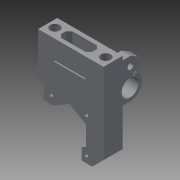
# Autodesk Inventor part: x-end-motor
Saved by Autodesk Inventor 2015 (Build 190159000, 159)
## iProperties
Created: 2015-06-01
Part Number: x-end-motor
Material: Generic
Document SubType Name: Modeling
Designer: X
Density: 1 g/cm^3
Appearance: Default
Author: X
Autodesk Inventor part; units mm, degrees
ref_plane "YZ Plane" through (0, 0, 0) normal (1, 0, 0) x (0, 1, 0)
ref_plane "XZ Plane" through (0, 0, 0) normal (0, 1, 0) x (-1, 0, 0)
ref_plane "XY Plane" through (0, 0, 0) normal (0, 0, 1) x (1, 0, 0)
sketch "Sketch1" plane through (0, 0, 0) normal (0, 1, 0) x (-1, 0, 0)
  line L0 (0, 0) -> (58, 0)
  line L1 (58, 0) -> (58, -81.5)
  line L2 (58, -81.5) -> (0, -81.5)
  line L3 (0, -81.5) -> (0, 0)
  dimension "d0" = 81.5
  dimension "d1" = 58
  constraints: 8 end point, 2 parallel, 1 horizontal, 1 perpendicular
  measures "d0" distance of L0.end L1.end
  measures "d1" distance between parallel lines of L3 L1
extrude "Extrusion1" add sketch "Sketch1" along normal blind 35
sketch "Sketch2" plane through (0, 35, 0) normal (0, 1, 0) x (1, 0, 0)
  line L0 (-30.25, 43.5) -> (-44.9724, 52)
  line L1 (-44.9724, 52) -> (-44.9724, 69)
  line L2 (-44.9724, 69) -> (-30.25, 77.5)
  line L3 (-30.25, 77.5) -> (-15.5276, 69)
  line L4 (-15.5276, 69) -> (-15.5276, 52)
  line L5 (-15.5276, 52) -> (-30.25, 43.5)
  line L6 (-58, 81.5) -> (-58, 0) projected
  line L7 (0, 81.5) -> (-58, 81.5) projected
  line L8 (-44.9724, 52) -> (-53, 52)
  line L9 (-19.25, 81.5) -> (-19.25, 71.1491)
  line L10 (0, 0) -> (0, 81.5) projected
  line L11 (-53, 52) -> (-53, 39.5)
  line L12 (-53, 39.5) -> (-58, 39.5)
  line L13 (-58, 39.5) -> (-58, 81.5)
  point P0 (-30.25, 60.5)
  dimension "d4" = 17
  dimension "d5" = 38
  dimension "d6" = 27.75
  dimension "d7" = 19.25
  dimension "d24" = 12.5
  dimension "d25" = 5
  constraints: 22 end point, 3 point on line, 2 perpendicular, 2 vertical, 1 parallel, 13 other
  measures "d4" distance of L3.end L4.end
  measures "d5" distance from line of L7 L0.start
  measures "d6" distance from line of L6 L0.start
  measures "d7" distance between parallel lines of L10 L9
  measures "d24" distance of L8.end L11.end
  measures "d25" distance of L11.end L12.end
extrude "Extrusion2" cut sketch "Sketch2" against normal through all
sketch "Sketch3" plane through (0, 0, 0) normal (1, 0, 0) x (0, 0, -1)
  line L0 (81.5, 0) -> (0, 0)
  line L1 (0, 0) -> (0, 17)
  line L2 (81.5, 17) -> (81.5, 0)
  line L3 (0, 0) -> (0, 35) projected
  line L4 (15.5, 30.8564) -> (19.5, 23.9282)
  line L5 (15.5, 17) -> (7.5, 17)
  line L6 (3.5, 23.9282) -> (7.5, 30.8564)
  line L7 (7.5, 30.8564) -> (15.5, 30.8564)
  line L8 (3.5, 23.9282) -> (3.5, 17)
  line L9 (19.5, 23.9282) -> (19.5, 17)
  circle A0 centre (27.7462, 23.5) radius 7.5
  circle A1 centre (27.7462, 23.5) radius 10.5
  line L10 (38.2462, 23.5) -> (38.2462, 17)
  line L11 (0, 17) -> (24.0046, 17)
  line L12 (31.4879, 17) -> (81.5, 17)
  point P0 (11.5, 23.9282)
  dimension "d10" = 17
  dimension "d11" = 3
  dimension "d12" = 15
  dimension "d13" = 6.5
  dimension "d14" = 3.5
  dimension "d15" = 8
  constraints: 24 end point, 7 perpendicular, 4 point on circle, 3 collinear, 3 parallel, 3 point on line, 2 centre point, 1 horizontal, 1 tangent, 9 other
  measures "d10" distance of L2.start L0.start
  measures "d11" radial gap between concentric circles of A1 A0
  measures "d12" diameter of A0
  measures "d13" distance of L10.start L10.end
  measures "d14" distance between parallel lines of L3 L8
  measures "d15" distance of L6.end L4.start
extrude "Extrusion4" cut sketch "Sketch3" against normal through all contours L0 L1 L11 L5 A1 L12 L2 | L12 A1 L10 | L8 L6 L7 L4 A1 L11 L5 | A1 L12 A0 L11 L9 L4 | A1 L11 A0 L12 | L4 L9 A1 keep common part
sketch "Sketch4" plane through (-58, 0, 0) normal (0, 0, 1) x (1, 0, 0)
  line L0 (0, 17) -> (50, 17)
  line L1 (50, 17) -> (50, 30.8564)
  line L2 (50, 30.8564) -> (0, 30.8564)
  line L3 (0, 30.8564) -> (0, 17)
  line L4 (0, 17) -> (58, 17) projected
  line L5 (0, 0) -> (0, 17) projected
  line L6 (58, 17) -> (58, 23.9282) projected
  line L7 (58, 30.8564) -> (0, 30.8564) projected
  point P0 (58, 0)
  point P1 (0, 35)
  dimension "d21" = 8
  constraints: 8 end point, 3 collinear, 2 parallel, 1 horizontal, 1 perpendicular
  measures "d21" distance between parallel lines of L6 L1
extrude "Extrusion5" cut sketch "Sketch4" against normal up to surface (17.8017 mm away)
sketch "Sketch5" plane through (0, 17, -38.2462) normal (0, 1, 0) x (1, 0, 0)
  line L0 (-8, -20.4446) -> (-58, -20.4446) projected
  line L1 (-16, -20.4446) -> (-44, -20.4446)
  line L2 (-44, -20.4446) -> (-44, -21.4446)
  line L3 (-44, -21.4446) -> (-16, -21.4446)
  line L4 (-16, -21.4446) -> (-16, -20.4446)
  line L5 (-8, -20.4446) -> (-8, -22.7462) projected
  point P0 (0, -38.2462)
  dimension "d26" = 8
  dimension "d27" = 1
  dimension "d28" = 28
  constraints: 8 end point, 2 parallel, 1 horizontal, 1 perpendicular, 1 point on line
  measures "d26" distance between parallel lines of L5 L4
  measures "d27" distance of L1.end L2.end
  measures "d28" distance of L2.end L3.end
extrude "Extrusion6" cut sketch "Sketch5" against normal through all
sketch "Sketch6" plane through (-44.9724, 0, -52) normal (0, 0, -1) x (-1, 0, 0)
  line L0 (-25.7224, 13.5) -> (-3.7224, 13.5)
  line L1 (-3.7224, 13.5) -> (-3.7224, 3.5)
  line L2 (-3.7224, 3.5) -> (-25.7224, 3.5)
  line L3 (-25.7224, 3.5) -> (-25.7224, 13.5)
  line L4 (-14.7224, 17) -> (-14.7224, 0) projected
  line L5 (-25.7224, 13.5) -> (-3.7224, 3.5) construction
  line L6 (-3.7224, 13.5) -> (-25.7224, 3.5) construction
  point P0 (-44.9724, 0)
  point P1 (-14.7224, 8.5)
  point P2 (-14.7224, 35)
  dimension "d31" = 10
  dimension "d32" = 22
  constraints: 12 end point, 3 midpoint, 2 parallel, 1 horizontal, 1 perpendicular
  measures "d31" distance of L0.end L1.end
  measures "d32" distance of L1.end L2.end
extrude "Extrusion7" cut sketch "Sketch6" against normal through all
sketch "Sketch7" plane through (-58, 0, 0) normal (0, 0, 1) x (1, 0, 0)
  line L0 (38.75, 3.5) -> (41.5, 6.25)
  line L1 (41.5, 6.25) -> (41.5, 10.75)
  line L2 (41.5, 10.75) -> (38.75, 13.5)
  line L3 (27.75, 3.5) -> (27.75, 13.5) construction
  line L4 (16.75, 13.5) -> (38.75, 13.5) construction
  line L5 (38.75, 13.5) -> (27.75, 13.5)
  line L6 (38.75, 3.5) -> (27.75, 3.5)
  line L7 (16.75, 3.5) -> (38.75, 3.5) projected
  line L8 (27.75, 8.5) -> (41.5, 8.5) construction
  line L9 (16.75, 3.5) -> (14, 6.25)
  line L10 (14, 6.25) -> (14, 10.75)
  line L11 (14, 10.75) -> (16.75, 13.5)
  line L12 (38.75, 13.5) -> (16.75, 13.5) construction
  line L13 (16.75, 13.5) -> (27.75, 13.5)
  line L14 (16.75, 3.5) -> (27.75, 3.5)
  point P0 (58, 0)
  dimension "d39" = 13.75
  dimension "d40" = 135
  dimension "d41" = 2.75
  constraints: 26 end point, 5 symmetric about line, 3 midpoint, 2 collinear, 2 point on line, 1 perpendicular, 1 other
  measures "d39" distance between parallel lines of L1 L3
  measures "d40" angle of L0 L6
  measures "d41" distance from line of L1 L0.start
extrude "Extrusion9" cut sketch "Sketch7" against normal blind 41.5
sketch "Sketch8" plane through (0, 17, -38.2462) normal (0, 1, 0) x (1, 0, 0)
  line L0 (-46.515, 6.0938) -> (-15.515, 6.0938) construction
  line L1 (-15.515, 6.0938) -> (-15.515, 37.0938) construction
  line L2 (-53, 13.7538) -> (-53, 1.2538) construction
  line L3 (-44.9724, 13.7538) -> (-53, 13.7538) construction
  point P0 (0, -38.2462)
  dimension "d45" = 31
  dimension "d46" = 31
  dimension "d47" = 6.485
  dimension "d48" = 7.66
  constraints: 4 end point, 1 horizontal, 1 perpendicular
  measures "d45" distance of L0.start L0.end
  measures "d46" distance of L1.end L0.end
  measures "d47" distance from line of L2 L0.start
  measures "d48" distance from line of L3 L0.start
hole "Hole1" at (-46.515, 17, -44.34) at (-15.515, 17, -44.34) at (-15.515, 17, -75.34) direction (0, -1, 0) diameter 3.6 end through all counterbore diameter 6.2 counterbore depth 3.5
sketch "Sketch9" plane through (-58, 0, 0) normal (0, 0, 1) x (1, 0, 0)
  line L0 (0, 0) -> (0, 17) construction
  line L1 (0, 8.5) -> (58, 8.5) construction
  line L2 (58, 0) -> (58, 17) construction
  line L3 (58, 0) -> (0, 0) construction
  point P0 (51.5, 8.5)
  point P1 (6.5, 8.5)
  point P2 (0, 35)
  point P3 (58, 35)
  dimension "d56" = 45
  dimension "d57" = 8.5
  dimension "d58" = 6.5
  constraints: 2 end point, 2 midpoint, 2 point on line, 1 horizontal
  measures "d56" distance of point (51.5, 8.5) point (6.5, 8.5)
  measures "d57" distance between parallel lines of L3 L1
  measures "d58" distance from line of L0 point (6.5, 8.5)
hole "Hole2" at (-6.5, 8.5, 0) at (-51.5, 8.5, 0) direction (0, 0, -1) diameter 8.5 depth 37
chamfer "Chamfer1" distance 10 angle 45 1 edges at (0, 8.5, -81.5)
hole "Hole3" at (0, 23.9282, -11.5) direction (-1, 0, 0) diameter 5.4 end through all
sketch "Sketch12" plane through (-8, 17, -17.8017) normal (-1, 0, 0) x (0, 0, 1)
  line L0 (8.5517, 10.8252) -> (10.8017, 6.9282)
  line L1 (10.8017, 6.9282) -> (8.5517, 3.0312)
  line L2 (8.5517, 3.0312) -> (4.0519, 3.0312)
  line L3 (4.0519, 3.0312) -> (1.8019, 6.9282)
  line L4 (1.8019, 6.9282) -> (4.0519, 10.8252)
  line L5 (4.0519, 10.8252) -> (8.5517, 10.8252)
  line L6 (2.3017, 13.8564) -> (10.3017, 13.8564) projected
  line L7 (10.3017, 13.8564) -> (14.3017, 6.9282) projected
  line L8 (10.8017, 6.9282) -> (14.3017, 6.9282) construction
  point P0 (17.8017, -17)
  point P1 (6.3018, 6.9282)
  dimension "d77" = 3.5
  dimension "d78" = 7.794
  constraints: 14 end point, 2 parallel, 1 horizontal, 13 other
  measures "d77" distance of L7.end L0.end
  measures "d78" distance between parallel lines of L2 L5
extrude "Extrusion10" cut sketch "Sketch12" against normal blind 5
sketch "Sketch13" plane through (-58, 0, -39.5) normal (-1, 0, 0) x (0, 0, 1)
  circle A0 centre (11.7538, 23.5) radius 7.5 projected
  line L0 (21.6983, 26.8698) -> (24, 30.8564) projected
  line L1 (18.874, 25.8564) -> (18.4972, 26.7827)
  line L2 (18.4972, 26.7827) -> (22.6151, 28.4577)
  line L3 (22.6151, 28.4577) -> (22.9919, 27.5314)
  line L4 (22.9919, 27.5314) -> (18.874, 25.8564)
  point P0 (39.5, 0)
  dimension "d81" = 1
  dimension "d82" = 1.675
  constraints: 8 end point, 2 perpendicular, 2 point on circle, 1 parallel, 1 point on line
  measures "d81" distance of L1.start L1.end
  measures "d82" vertical distance of L3.end L1.start
extrude "Extrusion11" cut sketch "Sketch13" against normal through all contours A0 L2 L0 L4 | L0 L3 L4
body "Solid1"
